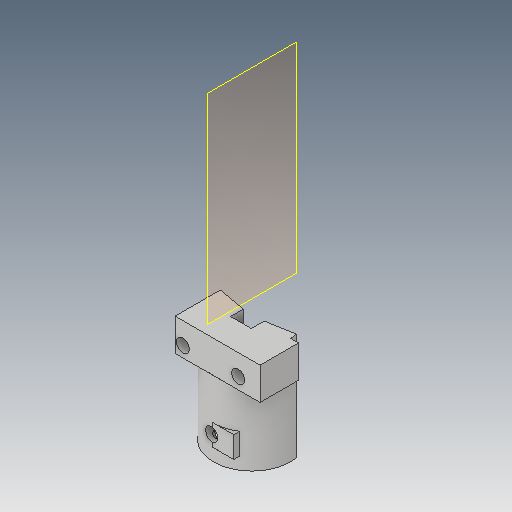
# Autodesk Inventor part: 30_CUBE_OpenSIM_Beamexpander_v2
Saved by Autodesk Inventor 2019 (Build 230136000, 136)
## iProperties
Created: 2019-10-22
Part Number: 30_CUBE_OpenSIM_Beamexpander_v2
Material: Generic
Document SubType Name: Modeling
Designer: diederichbenedict
Density: 1 g/cm^3
Appearance: Default
Author: diederichbenedict
Autodesk Inventor part; units mm, degrees
ref_plane "YZ Plane" through (0, 0, 0) normal (1, 0, 0) x (0, 1, 0)
ref_plane "XZ Plane" through (0, 0, 0) normal (0, 1, 0) x (-1, 0, 0)
ref_plane "XY Plane" through (0, 0, 0) normal (0, 0, 1) x (1, 0, 0)
ref_plane "Work Plane1" through (3.85, 70.2125, 8.85) normal (1, 0, 0) x (0, 0, 1)
sketch "Sketch1" plane through (3.85, 70.2125, 8.85) normal (1, 0, 0) x (0, 0, 1)
  line L0 (-8.85, 70.2125) -> (-17.05, 70.2125) construction
  line L1 (-17.05, 70.2125) -> (-17.05, 65.2125) construction
  line L2 (-8.85, 65.2125) -> (-17.05, 65.2125) construction
  line L3 (-8.85, 70.2125) -> (-8.85, 65.2125) construction
  arc A0 (-25.45, 97.2125) -> (-0.45, 97.2125) centre (-12.95, 114.7438) ccw construction
  arc A1 (-0.45, 99.2125) -> (-25.45, 99.2125) centre (-12.95, 81.6813) ccw construction
  line L4 (-0.45, 99.2125) -> (-0.45, 97.2125) construction
  line L5 (-25.45, 99.2125) -> (-25.45, 97.2125) construction
  line L6 (-12.95, -45.926) -> (-12.95, 188.756) construction
  line L7 (-10.1686, 64.1631) -> (-10.1686, 77.6475)
  line L8 (-10.1686, 77.6475) -> (-3.1244, 95.5852)
  line L9 (-3.1244, 100.8399) -> (-3.1244, 103.9225)
  line L10 (-3.1244, 103.9225) -> (1.3329, 103.9225)
  line L11 (1.3329, 103.9225) -> (1.3329, 64.1631)
  line L12 (1.3329, 64.1631) -> (-10.1686, 64.1631)
  arc A2 (-3.1244, 95.5852) -> (-0.45, 97.2125) centre (-12.95, 114.7438) ccw
  arc A3 (-0.45, 99.2125) -> (-3.1244, 100.8399) centre (-12.95, 81.6813) ccw
  line L13 (-0.45, 97.2125) -> (-0.45, 99.2125)
  constraints: 20 end point, 10 point on circle, 6 vertical, 4 centre point, 3 concentric, 3 perpendicular, 10 other
revolve "Revolution1" add sketch "Sketch1" angle 200 mid plane about axis through (3.85, 116.1385, -4.1) along (0, -1, 0)
sketch "Sketch2" plane through (3.85, 6.0495, -4.1) normal (0, 1, 0) x (1, 0, 0)
  circle A0 centre (0, 0) radius 2.8472 projected
  line L0 (-3.85, -4.1) -> (3.85, -4.1) projected
  line L1 (3.85, -4.1) -> (3.85, 4.1) projected
  line L2 (3.85, 4.1) -> (-3.85, 4.1) projected
  line L3 (-3.85, 4.1) -> (-3.85, -4.1) projected
  line L4 (-3.55, -3.8) -> (3.55, -3.8)
  line L5 (3.55, -3.8) -> (3.55, 3.8)
  line L6 (3.55, 3.8) -> (-3.55, 3.8)
  line L7 (-3.55, 3.8) -> (-3.55, -3.8)
  dimension "d1" = 0.3
  constraints: 8 end point, 3 other
  measures "d1" distance between parallel lines of L3 L7
extrude "Extrusion1" cut sketch "Sketch2" against normal through all contours A0 | L3 L2 L1 L0 | L7 L6 L5 L4
sketch "Sketch3" plane through (3.85, 6.0495, -4.1) normal (0, 1, 0) x (1, 0, 0)
  arc A0 (-14.0659, 2.4802) -> (14.0659, 2.4802) centre (0, 0) ccw projected
  line L0 (-14.2797, -0.3038) -> (-14.2797, -14.2829)
  line L1 (-14.2797, -0.3038) -> (-0.3006, -0.3038) construction
  line L2 (-14.2797, -14.2829) -> (0, -14.2829)
  line L3 (14.2797, -0.3038) -> (14.2797, -14.2829)
  line L4 (14.2797, -14.2829) -> (0, -14.2829)
  line L5 (14.2797, -14.2829) -> (17.2797, -14.2829)
  line L6 (17.2797, -14.2829) -> (17.2797, 0)
  line L7 (17.2797, 0) -> (14.2797, 0)
  line L8 (14.2797, 0) -> (14.2797, -14.2829)
  point P0 (-3.85, -4.1)
  dimension "d4" = 90
  dimension "d11" = 3
  constraints: 18 end point, 3 perpendicular, 3 point on circle, 2 horizontal, 2 parallel, 1 vertical
  measures "d4" angle of L0 L1
  measures "d11" distance of L7.end L6.end
extrude "Extrusion2" add sketch "Sketch3" against normal blind 12
sketch "Sketch6" plane through (-10.4297, 6.0495, 10.1829) normal (0, 0, 1) x (1, 0, 0)
  line L0 (13.7983, -35.2418) -> (21.7983, -35.2418)
  line L1 (21.7983, -35.2418) -> (21.7983, -27.2418)
  line L2 (21.7983, -27.2418) -> (13.7983, -27.2418)
  line L3 (13.7983, -27.2418) -> (13.7983, -35.2418)
  line L4 (13.7983, -35.2418) -> (21.7983, -27.2418)
  line L5 (21.7983, -35.2418) -> (13.7983, -27.2418)
  circle A0 centre (13.4583, -31.2418) radius 1.4 projected
  point P0 (10.4297, -6.0495)
  point P1 (17.7983, -31.2418)
  dimension "d12" = 8
  dimension "d13" = 8
  constraints: 12 end point, 2 midpoint, 2 parallel, 1 horizontal, 1 perpendicular
  measures "d12" distance of L2.end L1.end
  measures "d13" distance of L1.end L0.end
extrude "Extrusion3" add sketch "Sketch6" against normal up to surface
sketch "Sketch7" plane through (-10.4297, 6.0495, 10.1829) normal (0, 0, 1) x (1, 0, 0)
  circle A0 centre (23.447, -7.7206) radius 1.4 construction
  circle A1 centre (2.8893, -7.9757) radius 1.4 construction
  circle A2 centre (13.4583, -31.2418) radius 1.4 construction
  circle A3 centre (13.4583, -31.2418) radius 2.4
  circle A4 centre (23.447, -7.7206) radius 2.4
  circle A5 centre (2.8893, -7.9757) radius 2.4
  point P0 (10.4297, -6.0495)
  dimension "d16" = 4.8
  dimension "d17" = 4.8
  dimension "d18" = 4.8
  constraints: 3 centre point, 3 coincident
  measures "d16" diameter of A3
  measures "d17" diameter of A4
  measures "d18" diameter of A5
extrude "Extrusion4" cut sketch "Sketch7" against normal blind 4
body "Solid1"
